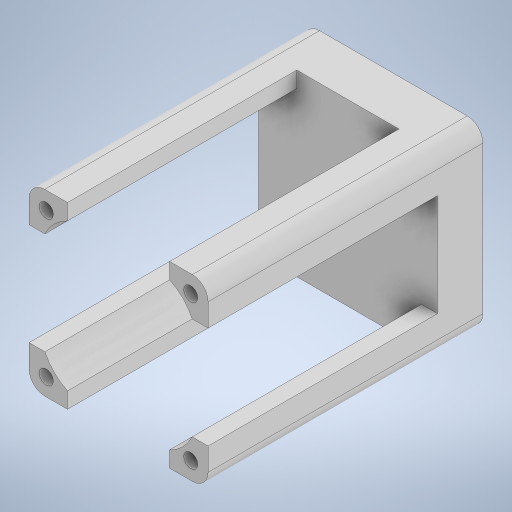
# Autodesk Inventor part: BackPlate
Saved by Autodesk Inventor 2024 (Build 280153000, 153)
## iProperties
Created: 2024-01-27
Part Number: BackPlate
Material: Generic
Document SubType Name: Modeling
Designer: Owner
Density: 1 g/cm^3
Appearance: Default
Author: Owner
Autodesk Inventor part; units mm, degrees
ref_plane "YZ Plane" through (0, 0, 0) normal (1, 0, 0) x (0, 1, 0)
ref_plane "XZ Plane" through (0, 0, 0) normal (0, 1, 0) x (-1, 0, 0)
ref_plane "XY Plane" through (0, 0, 0) normal (0, 0, 1) x (1, 0, 0)
sketch "Sketch1" plane through (0, 0, 0) normal (0, 0, 1) x (1, 0, 0)
  line L0 (0, 0) -> (114, 0)
  line L1 (114, 0) -> (114, 114)
  line L2 (114, 114) -> (0, 114)
  line L3 (0, 114) -> (0, 0)
  dimension "d0" = 114
  dimension "d1" = 114
  constraints: 8 end point, 2 parallel, 1 horizontal, 1 perpendicular
  measures "d0" distance of L1.end L2.end
  measures "d1" distance of L0.end L1.end
extrude "Extrusion1" add sketch "Sketch1" along normal blind 175
fillet "Fillet1" radius 10 1 edges at (0, 114, 87.5)
fillet "Fillet2" radius 10 3 edges at (114, 114, 87.5) (114, 0, 87.5) (0, 0, 87.5)
sketch "Sketch3" plane through (0, 0, 175) normal (0, 0, 1) x (1, 0, 0)
  circle A0 centre (11.038, 11.038) radius 4.5
  line L0 (10, 0) -> (104, 0) projected
  line L1 (0, 104) -> (0, 10) projected
  circle A1 centre (11.038, 102.962) radius 4.5
  circle A2 centre (102.962, 102.962) radius 4.5
  circle A3 centre (102.962, 11.038) radius 4.5
  line L2 (104, 114) -> (10, 114) projected
  line L3 (114, 10) -> (114, 104) projected
  point P0 (0, 0)
  dimension "d11" = 9
  dimension "d12" = 11.038
  dimension "d13" = 11.038
  dimension "d14" = 9
  dimension "d15" = 9
  dimension "d16" = 9
  dimension "d17" = 11.038
  dimension "d18" = 11.038
  dimension "d19" = 11.038
  dimension "d20" = 11.038
  dimension "d21" = 11.038
  dimension "d22" = 11.038
  constraints: 4 centre point
  measures "d11" diameter of A0
  measures "d12" distance from line of L0 A0.centre
  measures "d13" distance from line of L1 A0.centre
  measures "d14" diameter of A1
  measures "d15" diameter of A2
  measures "d16" diameter of A3
  measures "d17" distance from line of L2 A1.centre
  measures "d18" distance from line of L1 A1.centre
  measures "d19" distance from line of L3 A2.centre
  measures "d20" distance from line of L2 A2.centre
  measures "d21" distance from line of L3 A3.centre
  measures "d22" distance from line of L0 A3.centre
extrude "Extrusion3" cut sketch "Sketch3" against normal blind 146
sketch "Sketch6" plane through (0, 0, 175) normal (0, 0, 1) x (1, 0, 0)
  arc A0 (0, 10) -> (10, 0) centre (10, 10) ccw projected
  line L0 (0, 10) -> (0, 24.5)
  line L1 (0, 104) -> (0, 10) projected
  line L2 (0, 24.5) -> (10.13, 24.5)
  line L3 (10, 0) -> (24.5, 0)
  line L4 (10, 0) -> (104, 0) projected
  line L5 (24.5, 0) -> (24.5, 10.13)
  arc A1 (10.13, 24.5) -> (24.5, 10.13) centre (37.2744, 37.2744) ccw
  arc A2 (10, 114) -> (0, 104) centre (10, 104) ccw projected
  line L6 (10, 114) -> (24.5, 114)
  line L7 (104, 114) -> (10, 114) projected
  line L8 (24.5, 114) -> (24.5, 103.87)
  line L9 (0, 104) -> (0, 89.5)
  line L10 (0, 89.5) -> (10.13, 89.5)
  arc A3 (24.5, 103.87) -> (10.13, 89.5) centre (37.2744, 76.7256) ccw
  line L11 (104, 114) -> (89.5, 114)
  line L12 (89.5, 114) -> (89.5, 103.87)
  line L13 (114, 10) -> (114, 104) projected
  line L14 (114, 104) -> (114, 89.5)
  line L15 (114, 89.5) -> (114, 99.63)
  arc A4 (103.87, 89.5) -> (89.5, 103.87) centre (76.7256, 76.7256) ccw
  line L16 (103.87, 89.5) -> (114, 89.5)
  line L17 (114, 10) -> (114, 24.5)
  line L18 (114, 24.5) -> (103.87, 24.5)
  line L19 (104, 0) -> (89.5, 0)
  line L20 (89.5, 0) -> (89.5, 10.13)
  arc A5 (89.5, 10.13) -> (103.87, 24.5) centre (76.7256, 37.2744) ccw
  point P0 (0, 0)
  dimension "d30" = 14.5
  dimension "d31" = 10.13
  dimension "d32" = 14.5
  dimension "d33" = 10.13
  dimension "d34" = 30
  dimension "d35" = 14.5
  dimension "d36" = 10.13
  dimension "d37" = 14.5
  dimension "d38" = 10.13
  dimension "d39" = 30
  dimension "d40" = 14.5
  dimension "d41" = 10.13
  dimension "d42" = 14.5
  dimension "d44" = 30
  dimension "d45" = 10.13
  dimension "d46" = 14.5
  dimension "d47" = 10.13
  dimension "d48" = 14.5
  dimension "d49" = 10.13
  dimension "d50" = 30
  constraints: 34 end point, 9 point on line, 8 point on circle, 5 perpendicular, 4 centre point, 2 horizontal, 1 vertical
  measures "d30" distance of L0.start L0.end
  measures "d31" distance of L0.end L2.end
  measures "d32" distance of L3.start L3.end
  measures "d33" distance of L3.end L5.end
  measures "d34" radius of A1
  measures "d35" distance of L6.start L6.end
  measures "d36" distance of L6.end L8.end
  measures "d37" distance of L1.start L9.end
  measures "d38" distance of L9.end L10.end
  measures "d39" radius of A3
  measures "d40" distance of L7.start L11.end
  measures "d41" distance of L11.end L12.end
  measures "d42" distance of L13.end L14.end
  measures "d44" radius of A4
  measures "d45" distance of L16.start L14.end
  measures "d46" distance of L13.start L17.end
  measures "d47" distance of L17.end L18.end
  measures "d48" distance of L4.end L19.end
  measures "d49" distance of L19.end L20.end
  measures "d50" radius of A5
extrude "Extrusion5" cut sketch "Sketch6" against normal blind 146 contours L1 L10 A3 L8 L7 L12 A4 L16 L13 L18 A5 L20 L4 L5 A1 L2
equation "\"d13\" = d12"
equation "\"d17\" = d12"
equation "\"d18\" = d13"
equation "\"d19\" = d18"
equation "\"d20\" = d18"
equation "\"d21\" = d19"
equation "\"d22\" = d21"
equation "\"d33\" = d31"
body "Solid1"
